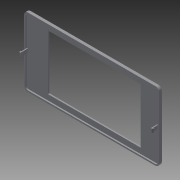
# Autodesk Inventor part: Slave Tablet Cover
Saved by Autodesk Inventor 2014 (Build 180170000, 170)
## iProperties
Created: 2015-08-04
Part Number: Slave Tablet Cover
Material: Generic
Document SubType Name: Modeling
Designer: Devon
Density: 1 g/cm^3
Appearance: Default
Author: Devon
Autodesk Inventor part; units mm, degrees
ref_plane "YZ Plane" through (0, 0, 0) normal (1, 0, 0) x (0, 1, 0)
ref_plane "XZ Plane" through (0, 0, 0) normal (0, 1, 0) x (-1, 0, 0)
ref_plane "XY Plane" through (0, 0, 0) normal (0, 0, 1) x (1, 0, 0)
sketch "Sketch1" plane through (0, 0, 0) normal (0, 0, 1) x (1, 0, 0)
  line L0 (-10.4542, 14.6019) -> (210.2083, 14.6019)
  line L1 (216.5583, 8.2519) -> (216.5583, -98.1106)
  line L2 (210.2083, -104.4606) -> (-10.4542, -104.4606)
  line L3 (-16.8042, -98.1106) -> (-16.8042, 8.2519)
  line L4 (99.877, 12.2207) -> (-10.4542, 12.2207)
  line L5 (-14.423, 8.2519) -> (-14.423, -44.9293)
  line L6 (99.877, 12.2207) -> (210.2083, 12.2207)
  line L7 (214.177, 8.2519) -> (214.177, -44.9293)
  line L8 (99.877, -102.0793) -> (210.2083, -102.0793)
  line L9 (214.177, -98.1106) -> (214.177, -44.9293)
  line L10 (99.877, -102.0793) -> (-10.4542, -102.0793)
  line L11 (-14.423, -98.1106) -> (-14.423, -44.9293)
  arc A0 (-10.4542, 14.6019) -> (-16.8042, 8.2519) centre (-10.4542, 8.2519) ccw
  arc A1 (216.5583, 8.2519) -> (210.2083, 14.6019) centre (210.2083, 8.2519) ccw
  arc A2 (210.2083, -104.4606) -> (216.5583, -98.1106) centre (210.2083, -98.1106) ccw
  arc A3 (-16.8042, -98.1106) -> (-10.4542, -104.4606) centre (-10.4542, -98.1106) ccw
  arc A4 (-10.4542, 12.2207) -> (-14.423, 8.2519) centre (-10.4542, 8.2519) ccw
  arc A5 (214.177, 8.2519) -> (210.2083, 12.2207) centre (210.2083, 8.2519) ccw
  arc A6 (210.2083, -102.0793) -> (214.177, -98.1106) centre (210.2083, -98.1106) ccw
  arc A7 (-14.423, -98.1106) -> (-10.4542, -102.0793) centre (-10.4542, -98.1106) ccw
  line L12 (99.877, 2.6957) -> (22.0895, 2.6957)
  line L13 (22.0895, 2.6957) -> (22.0895, -44.9293)
  line L14 (99.877, 2.6957) -> (182.427, 2.6957)
  line L15 (182.427, 2.6957) -> (182.427, -44.9293)
  line L16 (99.877, -92.5543) -> (182.427, -92.5543)
  line L17 (182.427, -92.5543) -> (182.427, -44.9293)
  line L18 (99.877, -92.5543) -> (22.0895, -92.5543)
  line L19 (22.0895, -92.5543) -> (22.0895, -44.9293)
  point P0 (0, 0)
  point P1 (-16.8042, 14.6019)
  point P2 (216.5583, -104.4606)
  point P3 (216.5583, 14.6019)
  point P4 (-16.8042, -104.4606)
  dimension "d0" = 233.3625
  dimension "d1" = 119.0625
  dimension "d9" = 6.35
  dimension "d10" = 3.9688
  dimension "d37" = 31.75
  dimension "d38" = 36.5125
  dimension "d39" = 9.525
  dimension "d40" = 9.525
  constraints: 40 end point, 16 point on circle, 16 tangent, 8 centre point, 8 point on line, 6 equal radius, 6 horizontal, 6 perpendicular, 2 parallel
  measures "d0" distance of point (216.558, -104.461) point (-16.804, -104.461)
  measures "d1" distance of point (216.558, 14.602) point (216.558, -104.461)
  measures "d9" radius of A0
  measures "d10" radius of A4
  measures "d37" distance of L7.end L15.end
  measures "d38" distance of L5.end L13.end
  measures "d39" distance of L4.start L12.start
  measures "d40" distance of L8.start L16.start
extrude "Extrusion5" add sketch "Sketch1" along normal blind 2.3813 contours L0 A1 L1 A2 L2 A3 L3 A0 | L6 A5 L7 L9 A6 L8 L10 A7 L11 L5 A4 L4
sketch "Sketch6" plane through (0, 0, 2.3813) normal (0, 0, 1) x (1, 0, 0)
  line L0 (210.2083, 14.6019) -> (-10.4542, 14.6019) projected
  arc A0 (-10.4542, 14.6019) -> (-16.8042, 8.2519) centre (-10.4542, 8.2519) ccw projected
  line L1 (-16.8042, 8.2519) -> (-16.8042, -98.1106) projected
  arc A1 (-16.8042, -98.1106) -> (-10.4542, -104.4606) centre (-10.4542, -98.1106) ccw projected
  line L2 (-10.4542, -104.4606) -> (210.2083, -104.4606) projected
  arc A2 (210.2083, -104.4606) -> (216.5583, -98.1106) centre (210.2083, -98.1106) ccw projected
  line L3 (216.5583, -98.1106) -> (216.5583, 8.2519) projected
  arc A3 (216.5583, 8.2519) -> (210.2083, 14.6019) centre (210.2083, 8.2519) ccw projected
  line L4 (99.877, 12.2207) -> (-10.4542, 12.2207)
  line L5 (-14.423, 8.2519) -> (-14.423, -44.9293)
  line L6 (99.877, 12.2207) -> (210.2083, 12.2207)
  line L7 (214.177, 8.2519) -> (214.177, -44.9293)
  line L8 (99.877, -102.0793) -> (210.2083, -102.0793)
  line L9 (214.177, -98.1106) -> (214.177, -44.9293)
  line L10 (99.877, -102.0793) -> (-10.4542, -102.0793)
  line L11 (-14.423, -98.1106) -> (-14.423, -44.9293)
  arc A4 (-10.4542, 12.2207) -> (-14.423, 8.2519) centre (-10.4542, 8.2519) ccw
  arc A5 (214.177, 8.2519) -> (210.2083, 12.2207) centre (210.2083, 8.2519) ccw
  arc A6 (210.2083, -102.0793) -> (214.177, -98.1106) centre (210.2083, -98.1106) ccw
  arc A7 (-14.423, -98.1106) -> (-10.4542, -102.0793) centre (-10.4542, -98.1106) ccw
  point P0 (0, 0)
  dimension "d47" = 3.9688
  constraints: 16 end point, 8 point on circle, 8 tangent, 4 centre point, 3 equal radius, 2 horizontal, 2 perpendicular
  measures "d47" radius of A4
extrude "Extrusion6" add sketch "Sketch6" along normal blind 2.3813
sketch "Sketch7" plane through (0, 0, 2.3813) normal (0, 0, 1) x (1, 0, 0)
  line L0 (-14.423, 8.2519) -> (-14.423, -98.1106) projected
  line L1 (214.177, -98.1106) -> (214.177, 8.2519) projected
  line L2 (-14.423, -44.9293) -> (-14.423, -41.7543)
  line L3 (-14.423, -41.7543) -> (-12.8355, -41.7543)
  line L4 (-12.8355, -41.7543) -> (-12.8355, -48.1043)
  line L5 (-12.8355, -48.1043) -> (-14.423, -48.1043)
  line L6 (-14.423, -48.1043) -> (-14.423, -44.9293)
  line L7 (214.177, -44.9293) -> (214.177, -41.7543)
  line L8 (214.177, -41.7543) -> (212.5895, -41.7543)
  line L9 (212.5895, -41.7543) -> (212.5895, -48.1043)
  line L10 (212.5895, -48.1043) -> (214.177, -48.1043)
  line L11 (214.177, -48.1043) -> (214.177, -44.9293)
  point P0 (0, 0)
  dimension "d50" = 3.175
  dimension "d51" = 1.5875
  dimension "d52" = 6.35
  dimension "d53" = 3.175
  dimension "d54" = 1.5875
  dimension "d55" = 6.35
  constraints: 20 end point, 4 perpendicular, 4 point on line, 2 collinear, 2 midpoint, 2 parallel
  measures "d50" distance of L2.start L2.end
  measures "d51" distance of L2.end L3.end
  measures "d52" distance of L3.end L4.end
  measures "d53" distance of L7.start L7.end
  measures "d54" distance of L7.end L8.end
  measures "d55" distance of L8.end L9.end
extrude "Extrusion7" add sketch "Sketch7" along normal blind 12.6937
sketch "Sketch8" plane through (214.177, -48.1043, 4.7625) normal (1, 0, 0) x (0, 0, -1)
  line L0 (0, 0) -> (-10.3124, 0) projected
  line L1 (-10.3124, 6.35) -> (-7.9248, 6.35)
  line L2 (-7.9248, 6.35) -> (-7.9248, 0)
  line L3 (-7.9248, 0) -> (-10.3124, 0)
  line L4 (-10.3124, 0) -> (-10.3124, 6.35)
  point P0 (4.7625, 48.1043)
  dimension "d58" = 2.3876
  constraints: 8 end point, 2 parallel, 1 horizontal, 1 perpendicular, 1 point on line
  measures "d58" distance of L2.end L3.end
extrude "Extrusion8" add sketch "Sketch8" along normal blind 1.5875
sketch "Sketch9" plane through (-14.423, -48.1043, 4.7625) normal (-1, 0, 0) x (0, 0, 1)
  line L0 (0, 0) -> (10.3124, 0) projected
  line L1 (10.3124, 6.35) -> (7.9248, 6.35)
  line L2 (7.9248, 6.35) -> (7.9248, 0)
  line L3 (7.9248, 0) -> (10.3124, 0)
  line L4 (10.3124, 0) -> (10.3124, 6.35)
  point P0 (-4.7625, 48.1043)
  dimension "d61" = 2.3876
  constraints: 8 end point, 2 parallel, 1 horizontal, 1 perpendicular, 1 point on line
  measures "d61" distance of L3.end L2.end
extrude "Extrusion9" add sketch "Sketch9" along normal blind 1.5875
sketch "Sketch10" plane through (212.5895, -41.7543, 2.3813) normal (0, 1, 0) x (1, 0, 0)
  line L0 (0, -12.6937) -> (3.175, -12.6937) projected
  line L1 (3.175, -10.3061) -> (3.175, -12.6937) projected
  line L2 (3.175, -10.3061) -> (1.5875, -10.3061)
  line L3 (1.5875, -10.3061) -> (1.5875, -12.6937)
  line L4 (1.5875, -12.6937) -> (3.175, -12.6937)
  line L5 (3.175, -12.6937) -> (3.175, -10.3061)
  line L6 (3.175, -11.4999) -> (3.175, -10.3061)
  line L7 (3.175, -10.903) -> (1.5875, -12.6937)
  point P0 (-212.5895, 2.3813)
  constraints: 12 end point, 3 midpoint, 2 parallel, 1 collinear, 1 horizontal, 1 perpendicular
split body "Split1" sketch "Sketch10" result one side removed curves L7 removed pieces at (215.6095, -43.871, 14.2128)
sketch "Sketch11" plane through (-14.423, -41.7543, 2.3813) normal (0, 1, 0) x (1, 0, 0)
  line L0 (-1.5875, -12.6937) -> (-1.5875, -10.3061) projected
  line L1 (1.5875, -12.6937) -> (-1.5875, -12.6937) projected
  line L2 (-1.5875, -10.3061) -> (0, -10.3061)
  line L3 (0, -10.3061) -> (0, -12.6937)
  line L4 (0, -12.6937) -> (-1.5875, -12.6937)
  line L5 (-1.5875, -12.6937) -> (-1.5875, -10.3061)
  line L6 (-1.5875, -11.4999) -> (-1.5875, -10.3061)
  line L7 (-1.5875, -10.903) -> (0, -12.6937)
  point P0 (14.423, 2.3813)
  constraints: 12 end point, 3 midpoint, 2 parallel, 1 collinear, 1 horizontal, 1 perpendicular
split body "Split2" sketch "Sketch11" result one side removed curves L7 removed pieces at (-15.8554, -43.871, 14.2128)
body "Solid2"
